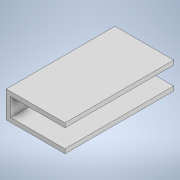
# Autodesk Inventor part: Lenkung
Saved by Autodesk Inventor 2020.3 (Build 243373010, 373A)
## iProperties
Created: 2020-11-21
Part Number: Lenkung
Material: Generisch
Document SubType Name: Modeling
Designer: Stefan
Density: 1 g/cm^3
Appearance: Vorgabe
Author: Stefan
Autodesk Inventor part; units mm, degrees
ref_plane "YZ Plane" through (0, 0, 0) normal (1, 0, 0) x (0, 1, 0)
ref_plane "XZ Plane" through (0, 0, 0) normal (0, 1, 0) x (-1, 0, 0)
ref_plane "XY Plane" through (0, 0, 0) normal (0, 0, 1) x (1, 0, 0)
sketch "Skizze2" plane through (0, 0, 0) normal (0, 1, 0) x (-1, 0, 0)
  line L0 (75, 150) -> (-75, 150)
  line L1 (-75, 150) -> (-75, -150)
  line L2 (-75, -150) -> (75, -150)
  line L3 (75, -150) -> (75, 150)
  point P0 (0, 0)
  dimension "d4" = 150
  dimension "d5" = 300
  dimension "d6" = 150
  dimension "d7" = 75
  constraints: 8 end point, 2 parallel, 1 horizontal, 1 perpendicular
  measures "d4" distance of L2.end L1.end
  measures "d5" distance of L2.end L0.start
  measures "d6" distance from line of point (0, 0) L2
  measures "d7" distance from line of L1 point (0, 0)
extrude "Extrusion2" add sketch "Skizze2" along normal blind 12
sketch "Skizze3" plane through (-75, 0, -150) normal (-1, 0, 0) x (0, 0, 1)
  line L0 (300, 0) -> (0, 0) projected
  line L1 (0, 0) -> (300, 0)
  line L2 (300, 0) -> (300, 74)
  line L3 (300, 74) -> (0, 74)
  line L4 (0, 74) -> (0, 0)
  point P0 (150, 0)
  dimension "d10" = 300
  dimension "d11" = 74
  constraints: 8 end point, 2 parallel, 1 horizontal, 1 perpendicular
  measures "d10" distance of L3.end L2.end
  measures "d11" distance of L2.end L1.end
extrude "Extrusion3" add sketch "Skizze3" along normal blind 12
sketch "Skizze4" plane through (-75, 0, -150) normal (1, 0, 0) x (0, 0, -1)
  line L0 (-300, 12) -> (-300, 74) projected
  line L1 (-300, 74) -> (0, 74)
  line L2 (0, 74) -> (0, 62)
  line L3 (0, 62) -> (-300, 62)
  line L4 (-300, 62) -> (-300, 74)
  point P0 (-150, 0)
  dimension "d14" = 300
  dimension "d15" = 12
  constraints: 8 end point, 2 parallel, 1 horizontal, 1 perpendicular
  measures "d14" distance of L2.end L3.end
  measures "d15" distance of L1.end L2.end
extrude "Extrusion4" add sketch "Skizze4" along normal blind 150
